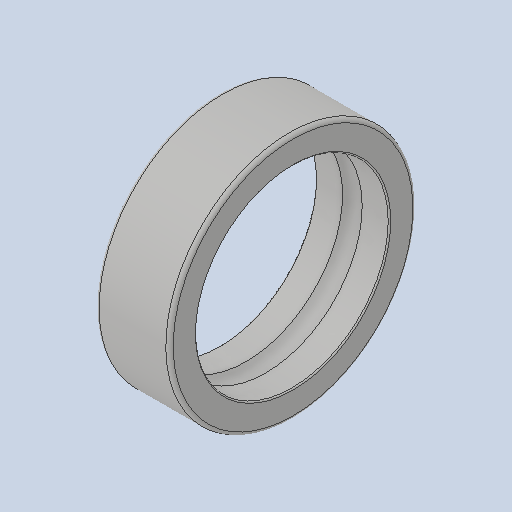
# Autodesk Inventor part: SKF_WBB1-8705_or
Saved by Autodesk Inventor 2024 (Build 280153000, 153)
## iProperties
Created: 2023-07-31
Part Number: SKF_WBB1-8705_or
Material: Generic
Catalog Web Link: www.cadenas.de
Description: BB1_001_101_or-Deep groove ball bearings
Vendor: SKF
Document SubType Name: Modeling
Designer: psAdmin
Manufacturer: SKF
Mass: 0.0899103 g
Surface Area: 2.26501 cm^2
Volume: 0.0899103 cm^3
Density: 1 g/cm^3
Appearance: PSOLRGB-175-175-175
Category: PARTsolutions
Company: SKF
PSOL_IDENT_0: {$CADENAS_DATA/23d-libs/skf/bearings_units_and_housings/ball_bearings/deep_groove_ball_bearings/part
PSOL_IDENT_1: s/bb1_001_101_or.prj},183 {VTYP=3D},{NB=SKF_WBB1-8705_or},{LINA=SKF_WBB1-8705_or},{NN=BB1_001_101_or
PSOL_IDENT_2: },{DATE=25.11.2022 05:56:16},{GEOMDATE=21.11.2022 10:24:00},{VERSION=},{LINEID=21100},{WBVAR=},{WBNU
PSOL_IDENT_3: MERIC=}  {NB=SKF_WBB1-8705_or},{LINA=SKF_WBB1-8705_or},{KT=DUMMY},{DESIGNATION=WBB1-8705},{R12=0.15}
PSOL_IDENT_4: ,{DD=5.000},{D=10.000},{B=3.000},{C=},{CX=},{CXX=},{CA=0.000},{XXVARIANT=},{XXDESIGN=Single row stai
PSOL_IDENT_5: nless steel},{XXSEALING=No seals},{DESIGN=dgbbw},{DESIGNIR=dgbbw},{VARIANT=},{DD1=6.00},{DD2=},{DD2X=
PSOL_IDENT_6: },{DD2A=0.00},{D1=7.80},{D1X=0.00},{D2=},{D2A=0.00},{D3=},{D3X=},{D3A=0.000},{D4=},{HH=0.000},{BB=0.
PSOL_IDENT_7: 000},{BBX=},{BBA=0.000},{FF=},{R0MAX=0.000},{R0=0.000},{PITCH=6.90},{DW=1.200},{DDAMIN=5.900},{DDAMA
PSOL_IDENT_8: X=0.000},{DDBMIN=0.000},{DDBMAX=0.000},{DBMIN=0.000},{DAMAX=8.800},{BBAMIN=0.000},{CAMAX=0.000},{RAM
PSOL_IDENT_9: AX=0.150},{LOAD1=0.247},{LOAD2=0.085},{LOAD3=0.004},{SPEED1=130000},{SPEED2=85000},{KR=0.015},{F0=7.
PSOL_IDENT_10: 600},{Z=8},{II=1},{MASS=0.001},{BEARING=WBB1-8705},{RING=},{HELP=1.100},{HELP2=1.100},{DD1ALG=3.000}
PSOL_IDENT_11: ,{YALG=3.000},{PITCH1=6.900},{DW1=1.200},{YALG1=3.900},{HALG1=1.100},{SH=3.000},{CU=0.360},{HALG=0.5
PSOL_IDENT_12: },{B1=0},{SHIELDHELP=1},{D4A=0.000},{FFA=0.000},{RS1=},{HELP3=0},{SUPPRESS=0}
NB: SKF_WBB1-8705_or
NN: BB1_001_101_or
NT: Deep groove ball bearings
NBSYN: SKF_$DESIGNATION._or
LINA: SKF_WBB1-8705_or
CATALOG: SKF
DESIGNATION: WBB1-8705
R12: 0.15
DD: 5
D: 10
B: 3
XXDESIGN: Single row stainless steel
XXSEALING: No seals
DD1: 6
D1: 7.8
D1X: 0
HH: 0
BB: 0
R0MAX: 0
R0: 0
PITCH: 6.9
DW: 1.2
DDAMIN: 5.9
DDAMAX: 0
DDBMIN: 0
DDBMAX: 0
DBMIN: 0
DAMAX: 8.8
BBAMIN: 0
CAMAX: 0
RAMAX: 0.15
LOAD1: 0.247
LOAD2: 0.085
LOAD3: 0.004
SPEED1: 130000
SPEED2: 85000
KR: 0.015
F0: 7.6
Z: 8
II: 1
MASS: 0.001
BEARING: WBB1-8705
HELP3: 0
SUPPRESS: 0
SUPPLIER: SKF
ARTICLENO: SKF_WBB1-8705_or
BOMINFO: SKF_WBB1-8705_or
CREATOR: CADENAS GmbH
Title: SKF_WBB1-8705_or
Author: Cadenas PARTsolutions
Comments: Deep groove ball bearings
Autodesk Inventor part; units mm, degrees
sketch "Sketch_7" plane through (0, 0, 0) normal (0, 0, 1) x (1, 0, 0)
  line L0 (3, 0) -> (-3, 0)
  arc A0 (0, 3.95) -> (0.05, 3.9) centre (0.05, 3.95) ccw
  line L1 (0.05, 3.9) -> (1.1031, 3.9)
  arc A1 (1.8969, 3.9) -> (1.1031, 3.9) centre (1.5, 3.45) ccw
  line L2 (1.8969, 3.9) -> (2.95, 3.9)
  arc A2 (2.95, 3.9) -> (3, 3.95) centre (2.95, 3.95) ccw
  line L3 (3, 3.95) -> (3, 4.85)
  arc A3 (3, 4.85) -> (2.85, 5) centre (2.85, 4.85) ccw
  line L4 (2.85, 5) -> (0.15, 5)
  arc A4 (0.15, 5) -> (0, 4.85) centre (0.15, 4.85) ccw
  line L5 (0, 4.85) -> (0, 3.95)
  constraints: 12 end point, 10 point on circle, 5 centre point
revolve "Revolution1" add sketch "Sketch_7" angle 360 about axis through (3, 0, 0) along (1, 0, 0)
ref_plane "or_XY" through (0, 0, 0) normal (0, 0, 1) x (1, 0, 0)
ref_plane "or_YZ" through (0, 0, 0) normal (1, 0, 0) x (0, 1, 0)
ref_plane "or_ZX" through (0, 0, 0) normal (0, 1, 0) x (0, 0, 1)
body "Solid1"
